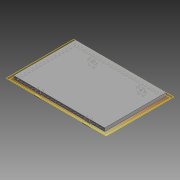
# Autodesk Inventor part: Deckel
Saved by Autodesk Inventor 2014 (Build 180170000, 170)
## iProperties
Created: 2016-07-21
Part Number: Deckel
Material: Generisch
Document SubType Name: Modeling
Designer: cem
Density: 1 g/cm^3
Appearance: Vorgabe
Author: cem
Autodesk Inventor part; units mm, degrees
ref_plane "YZ Plane" through (0, 0, 0) normal (1, 0, 0) x (0, 1, 0)
ref_plane "XZ Plane" through (0, 0, 0) normal (0, 1, 0) x (-1, 0, 0)
ref_plane "XY Plane" through (0, 0, 0) normal (0, 0, 1) x (1, 0, 0)
ref_plane "Arbeitsebene2" through (0, 0, 0.5) normal (0, 0, 1) x (1, 0, 0)
sketch "Skizze2" plane through (0, 0, 0.5) normal (0, 0, 1) x (1, 0, 0)
  line L0 (1.1, 14.6) -> (1.1, 13.85) projected
  line L1 (1.1, 13.85) -> (20.85, 13.85) projected
  line L2 (20.85, 13.85) -> (20.85, -13.85) projected
  line L3 (20.85, -13.85) -> (-20.85, -13.85) projected
  line L4 (-20.85, -13.85) -> (-20.85, 13.85) projected
  line L5 (-20.85, 13.85) -> (-7.4, 13.85) projected
  line L6 (-7.4, 13.85) -> (-7.4, 14.6) projected
  line L7 (-21.6, 14.6) -> (-7.4, 14.6) projected
  line L8 (-21.6, -14.6) -> (-21.6, 14.6) projected
  line L9 (21.6, -14.6) -> (-21.6, -14.6) projected
  line L10 (21.6, 14.6) -> (21.6, -14.6) projected
  line L11 (1.1, 14.6) -> (21.6, 14.6) projected
  line L12 (-21.6, 14.6) -> (21.6, 14.6)
  line L13 (21.6, 14.6) -> (21.6, -14.6)
  line L14 (21.6, -14.6) -> (-21.6, -14.6)
  line L15 (-21.6, -14.6) -> (-21.6, 14.6)
  point P0 (0, 0)
  constraints: 8 end point, 2 parallel, 1 horizontal, 1 perpendicular
extrude "Deckel" add sketch "Skizze2" along normal blind 1.5
sketch "Skizze3" plane through (0, 0, 0.5) normal (0, 0, -1) x (-1, 0, 0)
  line L0 (21.6, 14.6) -> (21.6, -14.6) projected
  line L1 (-21.6, 14.6) -> (21.6, 14.6) projected
  line L2 (-21.6, -14.6) -> (-21.6, 14.6) projected
  line L3 (21.6, -14.6) -> (-21.6, -14.6) projected
  line L4 (-1.1, 13.85) -> (-1.1, 13.1) projected
  line L5 (-20.1, 13.1) -> (-1.1, 13.1) projected
  line L6 (-20.1, -13.1) -> (-20.1, 13.1) projected
  line L7 (20.1, -13.1) -> (-20.1, -13.1) projected
  line L8 (20.1, 13.1) -> (20.1, -13.1) projected
  line L9 (7.4, 13.1) -> (20.1, 13.1) projected
  line L10 (7.4, 13.1) -> (7.4, 13.85) projected
  line L11 (20.85, 13.85) -> (7.4, 13.85) projected
  line L12 (20.85, -13.85) -> (20.85, 13.85) projected
  line L13 (-20.85, -13.85) -> (20.85, -13.85) projected
  line L14 (-20.85, 13.85) -> (-20.85, -13.85) projected
  line L15 (-1.1, 13.85) -> (-20.85, 13.85) projected
  line L16 (20.75, 13.75) -> (20.75, -13.75)
  line L17 (20.75, -13.75) -> (-20.75, -13.75)
  line L18 (-20.75, -13.75) -> (-20.75, 13.75)
  line L19 (-20.75, 13.75) -> (20.75, 13.75)
  point P0 (0, 0)
  dimension "d3" = 0.1
  constraints: 8 end point, 3 other
  measures "d3" distance between parallel lines of L19 L15
ref_plane "Führungsabstand" through (0, 0, 0.1) normal (0, 0, 1) x (1, 0, 0)
extrude "Führung" add sketch "Skizze3" along normal up to surface (0.4 mm away) contours L19 L10 L9 L8 L7 L6 L5 L4 | L4 L5 L6 L7 L8 L9 L10 L19 L16 L17 L18
sketch "Skizze6" plane through (20.75, -13.75, 0.1) normal (0, 0, -1) x (-1, 0, 0)
  line L0 (33.85, 26.85) -> (30.85, 26.85) projected
  line L1 (32.35, 27.8924) -> (32.35, 24.8924) construction
  line L2 (31.15, 26.65) -> (33.55, 26.65)
  line L3 (33.55, 26.65) -> (33.55, 25.45)
  line L4 (33.55, 25.45) -> (31.15, 25.45)
  line L5 (31.15, 25.45) -> (31.15, 26.65)
  point P0 (20.75, 13.75)
  point P1 (32.35, 26.85)
  dimension "d20" = 0.2
  dimension "d21" = 0.3
  dimension "d22" = 1.2
  constraints: 10 end point, 2 parallel, 2 perpendicular, 1 horizontal, 1 midpoint, 1 point on line, 1 other
  measures "d20" distance between parallel lines of L0 L2
  measures "d21" distance from line of L5 L0.end
  measures "d22" distance between parallel lines of L4 L2
ref_plane "Arbeitsebene7" through (-10.1, 13.1, -3) normal (0, 0, 1) x (1, 0, 0)
extrude "Schnapparm" add sketch "Skizze6" along normal up to surface (3.1 mm away)
sketch "Skizze7" plane through (-12.8, 12.9, 0.1) normal (0, 1, 0) x (1, 0, 0)
  line L0 (0, 3.1) -> (2.4, 3.1) projected
  line L1 (0, 0) -> (0, 3.1) projected
  line L2 (-0.3, 1.6) -> (2.7, 1.6) projected
  line L3 (-0.3, 3.4) -> (-0.3, 1.6) projected
  line L4 (2.7, 1.6) -> (2.7, 3.4) projected
  line L5 (2.7, 3.4) -> (-0.3, 3.4) projected
  line L6 (2.4, 3.1) -> (0, 3.1)
  line L7 (0, 3.1) -> (0, 1.9)
  line L8 (0, 1.9) -> (2.4, 1.9)
  line L9 (2.4, 1.9) -> (2.4, 3.1)
  point P0 (12.8, 0.1)
  dimension "d25" = 0.3
  constraints: 8 end point, 2 parallel, 1 horizontal, 1 perpendicular, 1 point on line
  measures "d25" distance between parallel lines of L2 L8
extrude "Schnapper" add sketch "Skizze7" along normal blind 1 contours L0 L9 L8 L1
chamfer "SchnapperPhase" distance 1 distance2 1 1 edges at (-11.6, 13.9, -3) measured on face at (-11.6, 13.9, -2.5)
draft "SchnapperVerjüngung" angle 10 pull direction (0, 0, -1) fixed plane through (-3.4667, -5.2667, 0.1) normal (0, 0, -1) faces at (-12, 11.7, -0.9333)
mirror "Schnapper2" about plane through (0, 0, 0) normal (1, 0, 0) of "Schnapparm", "Schnapper", "SchnapperPhase", "SchnapperVerjüngung"
mirror "Schnapper3" about plane through (0, 0, 0) normal (0, 1, 0) of "Schnapparm", "Schnapper", "SchnapperPhase", "SchnapperVerjüngung", "Schnapper2"
sketch "Skizze9" plane through (0, 0, 0.5) normal (0, 0, -1) x (-1, 0, 0)
  line L0 (-21.6, 14.6) -> (21.6, 14.6) projected
  line L1 (-1.1, 13.85) -> (-1.1, 13.1) projected
  line L2 (-1.1, 14.6) -> (-1.1, 13.85) projected
  line L3 (7.4, 13.1) -> (7.4, 13.85) projected
  line L4 (7.4, 13.85) -> (7.4, 14.6) projected
  line L5 (-1, 14.6) -> (7.3, 14.6)
  line L6 (7.3, 14.6) -> (7.3, 13.1)
  line L7 (7.3, 13.1) -> (-1, 13.1)
  line L8 (-1, 13.1) -> (-1, 14.6)
  point P0 (0, 0)
  point P1 (3.15, 14.6)
  dimension "d32" = 0.1
  dimension "d33" = 0.1
  constraints: 8 end point, 2 parallel, 2 point on line, 1 horizontal, 1 midpoint, 1 perpendicular
  measures "d32" distance between parallel lines of L8 L2
  measures "d33" distance between parallel lines of L4 L6
extrude "USB" add sketch "Skizze9" along normal blind 1.8
